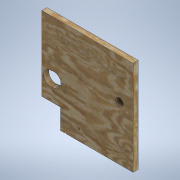
# Autodesk Inventor part: Shaft Mount with NEO mount
Saved by Autodesk Inventor 2020 (Build 240168000, 168)
## iProperties
Created: 2020-01-25
Part Number: Shaft Mount with NEO mount
Material: Wood (Maple)
Document SubType Name: Modeling
Designer: 1cikaychapman
Density: 0.67 g/cm^3
Appearance: Plywood - Weathered
Author: 1cikaychapman
Autodesk Inventor part; units mm, degrees
ref_plane "YZ Plane" through (0, 0, 0) normal (1, 0, 0) x (0, 1, 0)
ref_plane "XZ Plane" through (0, 0, 0) normal (0, 1, 0) x (-1, 0, 0)
ref_plane "XY Plane" through (0, 0, 0) normal (0, 0, 1) x (1, 0, 0)
sketch "Neo Motor Mount" plane through (0, 0, 0) normal (0, 0, 1) x (1, 0, 0)
  line L0 (-30.6788, 181.9654) -> (-23.3726, 145.6169) construction
  line L1 (-43.3455, 180.5359) -> (-35.6081, 142.0424) construction
  arc A0 (-42.1579, 174.6277) -> (-41.2194, 169.9586) centre (-41.6886, 172.2931) ccw
  line L2 (-35.6081, 142.0424) -> (-32.6003, 127.0788) construction
  line L3 (-23.3726, 145.6169) -> (-20.1494, 129.5815) construction
  arc A1 (-35.0803, 139.4164) -> (-34.1417, 134.7473) centre (-34.611, 137.0818) ccw
  arc A2 (-21.6908, 137.25) -> (-22.6293, 141.9191) centre (-22.16, 139.5845) ccw
  line L4 (-35.0803, 139.4164) -> (-22.6293, 141.9191)
  line L5 (-34.1417, 134.7473) -> (-21.6908, 137.25)
  arc A3 (-77.3692, 167.55) -> (-76.4307, 162.8809) centre (-76.9, 165.2155) ccw
  arc A4 (-63.9797, 165.3836) -> (-64.9183, 170.0527) centre (-64.449, 167.7182) ccw
  arc A5 (-70.2916, 132.3387) -> (-69.3531, 127.6696) centre (-69.8223, 130.0042) ccw
  arc A6 (-56.9021, 130.1723) -> (-57.8406, 134.8414) centre (-57.3714, 132.5069) ccw
  line L6 (-70.2916, 132.3387) -> (-57.8406, 134.8414)
  line L7 (-69.3531, 127.6696) -> (-56.9021, 130.1723)
  line L8 (-77.3692, 167.55) -> (-64.9183, 170.0527)
  line L9 (-76.4307, 162.8809) -> (-63.9797, 165.3836)
  arc A7 (-28.7684, 172.4613) -> (-29.7069, 177.1304) centre (-29.2377, 174.7958) ccw
  line L10 (-42.1579, 174.6277) -> (-29.7069, 177.1304)
  line L11 (-41.2194, 169.9586) -> (-28.7684, 172.4613)
  line L12 (-45.711, 165.6236) -> (-40.743, 140.9077) construction
  line L13 (-58.0667, 162.6468) -> (-53.1939, 138.405) construction
  line L14 (-57.5073, 159.8642) -> (-45.1815, 162.9896)
  line L15 (-53.7533, 141.1877) -> (-41.4275, 144.3131)
  arc A8 (-57.5073, 159.8642) -> (-52.8309, 141.4216) centre (-55.6303, 150.5259) ccw
  arc A9 (-46.2915, 152.4) -> (-46.438, 153.0215) centre (-55.6303, 150.5259) ccw
  arc A10 (-49.53, 157.8411) -> (-51.2107, 158.9635) centre (-55.6303, 150.5259) ccw
  arc A11 (-52.747, 152.4) -> (-52.6427, 151.7743) centre (-43.3045, 153.6514) ccw
  arc A12 (-49.53, 160.8603) -> (-51.2107, 158.9635) centre (-43.3045, 153.6514) ccw
  arc A13 (-41.4275, 144.3131) -> (-46.1039, 162.7557) centre (-43.3045, 153.6514) ccw
  dimension "d55" = 4.7625
  dimension "d57" = 4.7625
  dimension "d58" = 4.7625
  dimension "d61" = 4.7625
  dimension "d62" = 4.7625
  dimension "d63" = 4.7625
  dimension "d64" = 4.7625
  dimension "d65" = 4.7625
  dimension "d67" = 24.7159
  measures "d55" diameter of A0
  measures "d57" diameter of A1
  measures "d58" diameter of A2
  measures "d61" diameter of A3
  measures "d62" diameter of A4
  measures "d63" diameter of A5
  measures "d64" diameter of A6
  measures "d65" diameter of A7
  measures "d67" vertical distance of L12.start L12.end
sketch "Sketch1" plane through (0, 0, 0) normal (0, 0, 1) x (1, 0, 0)
  line L0 (0, 0) -> (254, 0)
  line L1 (254, 0) -> (254, 355.6)
  line L2 (254, 355.6) -> (0, 355.6)
  line L3 (0, 355.6) -> (-88.9, 355.6)
  line L4 (-88.9, 355.6) -> (-88.9, 203.2)
  line L5 (0, 0) -> (-19.05, 0)
  line L6 (-19.05, 0) -> (-19.05, 76.2)
  line L7 (-19.05, 76.2) -> (-88.9, 76.2)
  line L8 (-88.9, 76.2) -> (-88.9, 203.2)
  circle A0 centre (226.06, 181.61) radius 3.3782
  dimension "d29" = 6.7564
  dimension "d0" = 254
  dimension "d1" = 355.6
  dimension "d17" = 88.9
  dimension "d18" = 69.85
  dimension "d19" = 76.2
  dimension "d21" = 6.7564
  dimension "d24" = 173.99
  dimension "d28" = 314.96
  constraints: 18 end point, 5 perpendicular, 3 horizontal, 1 centre point, 1 parallel
  measures "d0" distance of L1.end L2.end
  measures "d1" distance of L0.end L1.end
  measures "d17" distance of L2.end L3.end
  measures "d18" distance of L7.end L6.end
  measures "d19" distance of L6.end L5.end
  measures "d21" diameter of A0
  measures "d24" vertical distance of L1.end A0.centre
  measures "d28" distance from line of L4 A0.centre
extrude "Extrusion1" add sketch "Sketch1" along normal blind 19.05 contours L5 L6 L7 L8 L4 L3 L2 L1 L0 | A0
sketch "Sketch2" plane through (0, 0, 19.05) normal (0, 0, 1) x (1, 0, 0)
  line L0 (0, 0) -> (254, 0) projected
  line L1 (254, 0) -> (254, 355.6) projected
  point P0 (203.2, 203.2)
  dimension "d11" = 203.2
  dimension "d12" = 50.8
  measures "d11" distance from line of L0 point (203.2, 203.2)
  measures "d12" distance from line of L1 point (203.2, 203.2)
hole "Hole1" at (203.2, 203.2, 19.05) direction (0, 0, -1) diameter 28.575 end through all
sketch "Sketch3" plane through (0, 0, 19.05) normal (0, 0, 1) x (1, 0, 0)
  point P0 (0, 0)
sketch "Sketch4" plane through (0, 0, 19.05) normal (0, 0, 1) x (1, 0, 0)
  point P0 (0, 0)
sketch "Sketch5" plane through (0, 0, 0) normal (0, 0, -1) x (-1, 0, 0)
  circle A0 centre (-7.62, 325.12) radius 3.3782
  circle A1 centre (2.54, 133.35) radius 3.3782
  circle A2 centre (-50.8, 40.64) radius 3.3782
  line L0 (-254, 0) -> (-254, 355.6) projected
  line L1 (-254, 355.6) -> (88.9, 355.6) projected
  line L2 (88.9, 76.2) -> (19.05, 76.2) construction
  line L3 (19.05, 76.2) -> (19.05, 374.6855) construction
  line L4 (19.05, 76.2) -> (19.05, 0) construction
  line L5 (19.05, 0) -> (-254, 0) construction
  point P0 (0, 0)
  dimension "d29" = 6.7564
  dimension "d30" = 6.7564
  dimension "d31" = 6.7564
  dimension "d32" = 246.38
  dimension "d33" = 256.54
  dimension "d34" = 203.2
  dimension "d35" = 30.48
  dimension "d36" = 222.25
  dimension "d37" = 314.96
  dimension "d40" = 16.51
  dimension "d42" = 26.67
  dimension "d43" = 40.64
  dimension "d44" = 133.35
  dimension "d45" = 325.12
  dimension "d46" = 69.85
  constraints: 3 centre point, 2 end point, 1 perpendicular
  measures "d29" diameter of A0
  measures "d30" diameter of A1
  measures "d31" diameter of A2
  measures "d32" distance from line of A0.centre L0
  measures "d33" distance from line of L0 A1.centre
  measures "d34" distance from line of L0 A2.centre
  measures "d35" distance from line of L1 A0.centre
  measures "d36" distance from line of L1 A1.centre
  measures "d37" distance from line of L1 A2.centre
  measures "d40" distance from line of A1.centre L3
  measures "d42" distance from line of A0.centre L3
  measures "d43" distance from line of L5 A2.centre
  measures "d44" distance from line of A1.centre L5
  measures "d45" distance from line of A0.centre L5
  measures "d46" distance from line of L4 A2.centre
extrude "Extrusion2" cut sketch "Sketch5" against normal through all
sketch "Sketch6" plane through (0, 0, 19.05) normal (0, 0, 1) x (1, 0, 0)
  line L0 (-114.6965, 152.4) -> (136.1638, 152.4) construction
  line L1 (-88.9, 355.6) -> (-88.9, 76.2) construction
  line L2 (-88.9, 76.2) -> (-19.05, 76.2) construction
  circle A0 centre (203.2, 203.2) radius 14.2875 construction
  line L3 (-49.53, 152.4) -> (203.2, 203.2) construction
  line L4 (-49.53, 152.4) -> (-245.9533, 112.9179) construction
  line L5 (-49.53, 44.7746) -> (-49.53, 143.2108) construction
  line L6 (-49.53, 146.4424) -> (-49.53, 372.917) construction
  line L7 (-58.0667, 162.6468) -> (-53.1939, 138.405) construction
  line L8 (-45.711, 165.6236) -> (-40.743, 140.9077) construction
  arc A1 (-38.8574, 127.4068) -> (-47.5966, 179.1246) centre (-43.227, 153.2657) ccw
  arc A2 (-60.1251, 177.0076) -> (-51.3859, 125.2897) centre (-55.7555, 151.1486) ccw
  line L9 (-60.1251, 177.0076) -> (-47.5966, 179.1246)
  line L10 (-51.3859, 125.2897) -> (-38.8574, 127.4068)
  point P0 (0, 0)
  point P1 (-57.5073, 159.8642)
  point P2 (-45.1815, 162.9896)
  point P3 (-53.7533, 141.1877)
  point P4 (-41.4275, 144.3131)
  point P5 (-47.5966, 179.1246)
  dimension "d48" = 76.2
  dimension "d83" = 24.7159
  constraints: 18 end point, 8 point on line, 5 point on circle, 2 centre point, 2 vertical, 1 collinear, 1 horizontal, 1 midpoint
  measures "d48" distance between parallel lines of L0 L2
  measures "d83" vertical distance of L8.start L8.end
extrude "Extrusion4" cut sketch "Sketch6" against normal through all
body "Solid1"
